Autodesk Fusion 360 part; units mm, degrees
(part 2 of 5)
  line L872 (126.5346, -132.5769) -> (126.5481, -132.5904)
  line L873 (126.5481, -132.5904) -> (126.55, -132.6)
  line L874 (126.55, -132.6) -> (126.55, -134.1)
  line L875 (126.55, -134.1) -> (126.5481, -134.1096)
  line L876 (126.5481, -134.1096) -> (126.5346, -134.1231)
  line L877 (126.5346, -134.1231) -> (126.525, -134.125)
  line L878 (126.525, -134.125) -> (121.125, -134.125)
  line L879 (121.125, -134.125) -> (121.1154, -134.1231)
  line L880 (121.1154, -134.1231) -> (121.1019, -134.1096)
  line L881 (121.1019, -134.1096) -> (121.1, -134.1)
  line L882 (121.1, -134.1) -> (121.1, -132.6)
  line L883 (121.1, -132.6) -> (121.1019, -132.5904)
  line L884 (121.1019, -132.5904) -> (121.1154, -132.5769)
  line L885 (121.1154, -132.5769) -> (121.125, -132.575)
  line L886 (121.125, -132.575) -> (126.525, -132.575)
  line L887 (126.525, -132.575) -> (126.5346, -132.5769)
  line L888 (121.15, -132.625) -> (121.15, -134.075)
  line L889 (121.15, -134.075) -> (126.5, -134.075)
  line L890 (126.5, -134.075) -> (126.5, -132.625)
  line L891 (126.5, -132.625) -> (121.15, -132.625)
  line L892 (62.5173, -130.6479) -> (62.5309, -130.6614)
  line L893 (62.5309, -130.6614) -> (62.5328, -130.671)
  line L894 (62.5328, -130.671) -> (62.5328, -132.1593)
  line L895 (62.5328, -132.1593) -> (62.5309, -132.1688)
  line L896 (62.5309, -132.1688) -> (62.5173, -132.1824)
  line L897 (62.5173, -132.1824) -> (62.5078, -132.1843)
  line L898 (62.5078, -132.1843) -> (61.0195, -132.1843)
  line L899 (61.0195, -132.1843) -> (61.0099, -132.1824)
  line L900 (61.0099, -132.1824) -> (60.9964, -132.1688)
  line L901 (60.9964, -132.1688) -> (60.9945, -132.1593)
  line L902 (60.9945, -132.1593) -> (60.9945, -130.671)
  line L903 (60.9945, -130.671) -> (60.9964, -130.6614)
  line L904 (60.9964, -130.6614) -> (61.0099, -130.6479)
  line L905 (61.0099, -130.6479) -> (61.0195, -130.646)
  line L906 (61.0195, -130.646) -> (62.5078, -130.646)
  line L907 (62.5078, -130.646) -> (62.5173, -130.6479)
  line L908 (61.0445, -130.696) -> (61.0445, -132.1343)
  line L909 (61.0445, -132.1343) -> (62.4828, -132.1343)
  line L910 (62.4828, -132.1343) -> (62.4828, -130.696)
  line L911 (62.4828, -130.696) -> (61.0445, -130.696)
  line L912 (67.5775, -130.6479) -> (67.591, -130.6614)
  line L913 (67.591, -130.6614) -> (67.5929, -130.671)
  line L914 (67.5929, -130.671) -> (67.5929, -132.1593)
  line L915 (67.5929, -132.1593) -> (67.591, -132.1688)
  line L916 (67.591, -132.1688) -> (67.5775, -132.1824)
  line L917 (67.5775, -132.1824) -> (67.5679, -132.1843)
  line L918 (67.5679, -132.1843) -> (66.0796, -132.1843)
  line L919 (66.0796, -132.1843) -> (66.0701, -132.1824)
  line L920 (66.0701, -132.1824) -> (66.0565, -132.1688)
  line L921 (66.0565, -132.1688) -> (66.0546, -132.1593)
  line L922 (66.0546, -132.1593) -> (66.0546, -130.671)
  line L923 (66.0546, -130.671) -> (66.0565, -130.6614)
  line L924 (66.0565, -130.6614) -> (66.0701, -130.6479)
  line L925 (66.0701, -130.6479) -> (66.0796, -130.646)
  line L926 (66.0796, -130.646) -> (67.5679, -130.646)
  line L927 (67.5679, -130.646) -> (67.5775, -130.6479)
  line L928 (66.1046, -130.696) -> (66.1046, -132.1343)
  line L929 (66.1046, -132.1343) -> (67.5429, -132.1343)
  line L930 (67.5429, -132.1343) -> (67.5429, -130.696)
  line L931 (67.5429, -130.696) -> (66.1046, -130.696)
  line L932 (93.1758, -121.4205) -> (93.1894, -121.4341)
  line L933 (93.1894, -121.4341) -> (93.1913, -121.4436)
  line L934 (93.1913, -121.4436) -> (93.1913, -125.0155)
  line L935 (93.1913, -125.0155) -> (93.1894, -125.0251)
  line L936 (93.1894, -125.0251) -> (93.1758, -125.0386)
  line L937 (93.1758, -125.0386) -> (93.1663, -125.0405)
  line L938 (93.1663, -125.0405) -> (90.81, -125.0405)
  line L939 (90.81, -125.0405) -> (90.81, -125.9085)
  line L940 (90.81, -125.9085) -> (90.8081, -125.918)
  line L941 (90.8081, -125.918) -> (90.7946, -125.9316)
  line L942 (90.7946, -125.9316) -> (90.785, -125.9335)
  line L943 (90.785, -125.9335) -> (88.1311, -125.9335)
  line L944 (88.1311, -125.9335) -> (88.1311, -129.778)
  line L945 (88.1311, -129.778) -> (88.1311, -130.9686)
  line L946 (88.1311, -130.9686) -> (88.1292, -130.9782)
  line L947 (88.1292, -130.9782) -> (88.1157, -130.9917)
  line L948 (88.1157, -130.9917) -> (88.1061, -130.9936)
  line L949 (88.1061, -130.9936) -> (83.6413, -130.9936)
  line L950 (83.6413, -130.9936) -> (83.3436, -130.9936)
  line L951 (83.3436, -130.9936) -> (83.334, -130.9917)
  line L952 (83.334, -130.9917) -> (83.3205, -130.9782)
  line L953 (83.3205, -130.9782) -> (83.3186, -130.9686)
  line L954 (83.3186, -130.9686) -> (83.3186, -128.0171)
  line L955 (83.3186, -128.0171) -> (81.8803, -128.0171)
  line L956 (81.8803, -128.0171) -> (81.8803, -129.778)
  line L957 (81.8803, -129.778) -> (81.8784, -129.7876)
  line L958 (81.8784, -129.7876) -> (81.8649, -129.8011)
  line L959 (81.8649, -129.8011) -> (81.8553, -129.803)
  line L960 (81.8553, -129.803) -> (79.4741, -129.803)
  line L961 (79.4741, -129.803) -> (79.4645, -129.8011)
  line L962 (79.4645, -129.8011) -> (79.451, -129.7876)
  line L963 (79.451, -129.7876) -> (79.4491, -129.778)
  line L964 (79.4491, -129.778) -> (79.4491, -127.7194)
  line L965 (79.4491, -127.7194) -> (77.0928, -127.7194)
  line L966 (77.0928, -127.7194) -> (77.0833, -127.7175)
  line L967 (77.0833, -127.7175) -> (77.0697, -127.704)
  line L968 (77.0697, -127.704) -> (77.0678, -127.6944)
  line L969 (77.0678, -127.6944) -> (77.0678, -124.4202)
  line L970 (77.0678, -124.4202) -> (77.0697, -124.4106)
  line L971 (77.0697, -124.4106) -> (77.0833, -124.3971)
  line L972 (77.0833, -124.3971) -> (77.0928, -124.3952)
  line L973 (77.0928, -124.3952) -> (79.4491, -124.3952)
  line L974 (79.4491, -124.3952) -> (79.4491, -121.4436)
  line L975 (79.4491, -121.4436) -> (79.451, -121.4341)
  line L976 (79.451, -121.4341) -> (79.4645, -121.4205)
  line L977 (79.4645, -121.4205) -> (79.4741, -121.4186)
  line L978 (79.4741, -121.4186) -> (93.1663, -121.4186)
  line L979 (93.1663, -121.4186) -> (93.1758, -121.4205)
  line L980 (79.4991, -121.4686) -> (79.4991, -124.4202)
  line L981 (79.4991, -124.4202) -> (79.4972, -124.4298)
  line L982 (79.4972, -124.4298) -> (79.4836, -124.4433)
  line L983 (79.4836, -124.4433) -> (79.4741, -124.4452)
  line L984 (79.4741, -124.4452) -> (77.1178, -124.4452)
  line L985 (77.1178, -124.4452) -> (77.1178, -127.6694)
  line L986 (77.1178, -127.6694) -> (79.4741, -127.6694)
  line L987 (79.4741, -127.6694) -> (79.4836, -127.6713)
  line L988 (79.4836, -127.6713) -> (79.4972, -127.6848)
  line L989 (79.4972, -127.6848) -> (79.4991, -127.6944)
  line L990 (79.4991, -127.6944) -> (79.4991, -129.753)
  line L991 (79.4991, -129.753) -> (81.8303, -129.753)
  line L992 (81.8303, -129.753) -> (81.8303, -127.9921)
  line L993 (81.8303, -127.9921) -> (81.8322, -127.9825)
  line L994 (81.8322, -127.9825) -> (81.8458, -127.969)
  line L995 (81.8458, -127.969) -> (81.8553, -127.9671)
  line L996 (81.8553, -127.9671) -> (83.3436, -127.9671)
  line L997 (83.3436, -127.9671) -> (83.3532, -127.969)
  line L998 (83.3532, -127.969) -> (83.3667, -127.9825)
  line L999 (83.3667, -127.9825) -> (83.3686, -127.9921)
  line L1000 (83.3686, -127.9921) -> (83.3686, -130.9436)
  line L1001 (83.3686, -130.9436) -> (83.6413, -130.9436)
  line L1002 (83.6413, -130.9436) -> (88.0811, -130.9436)
  line L1003 (88.0811, -130.9436) -> (88.0811, -129.778)
  line L1004 (88.0811, -129.778) -> (88.0811, -125.9085)
  line L1005 (88.0811, -125.9085) -> (88.083, -125.8989)
  line L1006 (88.083, -125.8989) -> (88.0965, -125.8854)
  line L1007 (88.0965, -125.8854) -> (88.1061, -125.8835)
  line L1008 (88.1061, -125.8835) -> (90.76, -125.8835)
  line L1009 (90.76, -125.8835) -> (90.76, -125.0155)
  line L1010 (90.76, -125.0155) -> (90.7619, -125.0059)
  line L1011 (90.7619, -125.0059) -> (90.7754, -124.9924)
  line L1012 (90.7754, -124.9924) -> (90.785, -124.9905)
  line L1013 (90.785, -124.9905) -> (93.1413, -124.9905)
  line L1014 (93.1413, -124.9905) -> (93.1413, -121.4686)
  line L1015 (93.1413, -121.4686) -> (79.4991, -121.4686)
  line L1016 (112.2258, -121.4205) -> (112.2394, -121.4341)
  line L1017 (112.2394, -121.4341) -> (112.2413, -121.4436)
  line L1018 (112.2413, -121.4436) -> (112.2413, -125.0155)
  line L1019 (112.2413, -125.0155) -> (112.2394, -125.0251)
  line L1020 (112.2394, -125.0251) -> (112.2258, -125.0386)
  line L1021 (112.2258, -125.0386) -> (112.2163, -125.0405)
  line L1022 (112.2163, -125.0405) -> (109.86, -125.0405)
  line L1023 (109.86, -125.0405) -> (109.86, -125.9085)
  line L1024 (109.86, -125.9085) -> (109.8581, -125.918)
  line L1025 (109.8581, -125.918) -> (109.8446, -125.9316)
  line L1026 (109.8446, -125.9316) -> (109.835, -125.9335)
  line L1027 (109.835, -125.9335) -> (107.1811, -125.9335)
  line L1028 (107.1811, -125.9335) -> (107.1811, -129.778)
  line L1029 (107.1811, -129.778) -> (107.1811, -130.9686)
  line L1030 (107.1811, -130.9686) -> (107.1792, -130.9782)
  line L1031 (107.1792, -130.9782) -> (107.1657, -130.9917)
  line L1032 (107.1657, -130.9917) -> (107.1561, -130.9936)
  line L1033 (107.1561, -130.9936) -> (102.6913, -130.9936)
  line L1034 (102.6913, -130.9936) -> (102.3936, -130.9936)
  line L1035 (102.3936, -130.9936) -> (102.384, -130.9917)
  line L1036 (102.384, -130.9917) -> (102.3705, -130.9782)
  line L1037 (102.3705, -130.9782) -> (102.3686, -130.9686)
  line L1038 (102.3686, -130.9686) -> (102.3686, -128.0171)
  line L1039 (102.3686, -128.0171) -> (100.9303, -128.0171)
  line L1040 (100.9303, -128.0171) -> (100.9303, -129.778)
  line L1041 (100.9303, -129.778) -> (100.9284, -129.7876)
  line L1042 (100.9284, -129.7876) -> (100.9149, -129.8011)
  line L1043 (100.9149, -129.8011) -> (100.9053, -129.803)
  line L1044 (100.9053, -129.803) -> (98.5241, -129.803)
  line L1045 (98.5241, -129.803) -> (98.5145, -129.8011)
  line L1046 (98.5145, -129.8011) -> (98.501, -129.7876)
  line L1047 (98.501, -129.7876) -> (98.4991, -129.778)
  line L1048 (98.4991, -129.778) -> (98.4991, -127.7194)
  line L1049 (98.4991, -127.7194) -> (96.1428, -127.7194)
  line L1050 (96.1428, -127.7194) -> (96.1333, -127.7175)
  line L1051 (96.1333, -127.7175) -> (96.1197, -127.704)
  line L1052 (96.1197, -127.704) -> (96.1178, -127.6944)
  line L1053 (96.1178, -127.6944) -> (96.1178, -124.4202)
  line L1054 (96.1178, -124.4202) -> (96.1197, -124.4106)
  line L1055 (96.1197, -124.4106) -> (96.1333, -124.3971)
  line L1056 (96.1333, -124.3971) -> (96.1428, -124.3952)
  line L1057 (96.1428, -124.3952) -> (98.4991, -124.3952)
  line L1058 (98.4991, -124.3952) -> (98.4991, -121.4436)
  line L1059 (98.4991, -121.4436) -> (98.501, -121.4341)
  line L1060 (98.501, -121.4341) -> (98.5145, -121.4205)
  line L1061 (98.5145, -121.4205) -> (98.5241, -121.4186)
  line L1062 (98.5241, -121.4186) -> (112.2163, -121.4186)
  line L1063 (112.2163, -121.4186) -> (112.2258, -121.4205)
  line L1064 (98.5491, -121.4686) -> (98.5491, -124.4202)
  line L1065 (98.5491, -124.4202) -> (98.5472, -124.4298)
  line L1066 (98.5472, -124.4298) -> (98.5336, -124.4433)
  line L1067 (98.5336, -124.4433) -> (98.5241, -124.4452)
  line L1068 (98.5241, -124.4452) -> (96.1678, -124.4452)
  line L1069 (96.1678, -124.4452) -> (96.1678, -127.6694)
  line L1070 (96.1678, -127.6694) -> (98.5241, -127.6694)
  line L1071 (98.5241, -127.6694) -> (98.5336, -127.6713)
  line L1072 (98.5336, -127.6713) -> (98.5472, -127.6848)
  line L1073 (98.5472, -127.6848) -> (98.5491, -127.6944)
  line L1074 (98.5491, -127.6944) -> (98.5491, -129.753)
  line L1075 (98.5491, -129.753) -> (100.8803, -129.753)
  line L1076 (100.8803, -129.753) -> (100.8803, -127.9921)
  line L1077 (100.8803, -127.9921) -> (100.8822, -127.9825)
  line L1078 (100.8822, -127.9825) -> (100.8958, -127.969)
  line L1079 (100.8958, -127.969) -> (100.9053, -127.9671)
  line L1080 (100.9053, -127.9671) -> (102.3936, -127.9671)
  line L1081 (102.3936, -127.9671) -> (102.4032, -127.969)
  line L1082 (102.4032, -127.969) -> (102.4167, -127.9825)
  line L1083 (102.4167, -127.9825) -> (102.4186, -127.9921)
  line L1084 (102.4186, -127.9921) -> (102.4186, -130.9436)
  line L1085 (102.4186, -130.9436) -> (102.6913, -130.9436)
  line L1086 (102.6913, -130.9436) -> (107.1311, -130.9436)
  line L1087 (107.1311, -130.9436) -> (107.1311, -129.778)
  line L1088 (107.1311, -129.778) -> (107.1311, -125.9085)
  line L1089 (107.1311, -125.9085) -> (107.133, -125.8989)
  line L1090 (107.133, -125.8989) -> (107.1465, -125.8854)
  line L1091 (107.1465, -125.8854) -> (107.1561, -125.8835)
  line L1092 (107.1561, -125.8835) -> (109.81, -125.8835)
  line L1093 (109.81, -125.8835) -> (109.81, -125.0155)
  line L1094 (109.81, -125.0155) -> (109.8119, -125.0059)
  line L1095 (109.8119, -125.0059) -> (109.8254, -124.9924)
  line L1096 (109.8254, -124.9924) -> (109.835, -124.9905)
  line L1097 (109.835, -124.9905) -> (112.1913, -124.9905)
  line L1098 (112.1913, -124.9905) -> (112.1913, -121.4686)
  line L1099 (112.1913, -121.4686) -> (98.5491, -121.4686)
  line L1100 (131.2758, -121.4205) -> (131.2894, -121.4341)
  line L1101 (131.2894, -121.4341) -> (131.2913, -121.4436)
  line L1102 (131.2913, -121.4436) -> (131.2913, -125.0155)
  line L1103 (131.2913, -125.0155) -> (131.2894, -125.0251)
  line L1104 (131.2894, -125.0251) -> (131.2758, -125.0386)
  line L1105 (131.2758, -125.0386) -> (131.2663, -125.0405)
  line L1106 (131.2663, -125.0405) -> (128.91, -125.0405)
  line L1107 (128.91, -125.0405) -> (128.91, -125.9085)
  line L1108 (128.91, -125.9085) -> (128.9081, -125.918)
  line L1109 (128.9081, -125.918) -> (128.8946, -125.9316)
  line L1110 (128.8946, -125.9316) -> (128.885, -125.9335)
  line L1111 (128.885, -125.9335) -> (126.2311, -125.9335)
  line L1112 (126.2311, -125.9335) -> (126.2311, -129.778)
  line L1113 (126.2311, -129.778) -> (126.2311, -130.9686)
  line L1114 (126.2311, -130.9686) -> (126.2292, -130.9782)
  line L1115 (126.2292, -130.9782) -> (126.2157, -130.9917)
  line L1116 (126.2157, -130.9917) -> (126.2061, -130.9936)
  line L1117 (126.2061, -130.9936) -> (121.7413, -130.9936)
  line L1118 (121.7413, -130.9936) -> (121.4436, -130.9936)
  line L1119 (121.4436, -130.9936) -> (121.434, -130.9917)
  line L1120 (121.434, -130.9917) -> (121.4205, -130.9782)
  line L1121 (121.4205, -130.9782) -> (121.4186, -130.9686)
  line L1122 (121.4186, -130.9686) -> (121.4186, -128.0171)
  line L1123 (121.4186, -128.0171) -> (119.9803, -128.0171)
  line L1124 (119.9803, -128.0171) -> (119.9803, -129.778)
  line L1125 (119.9803, -129.778) -> (119.9784, -129.7876)
  line L1126 (119.9784, -129.7876) -> (119.9649, -129.8011)
  line L1127 (119.9649, -129.8011) -> (119.9553, -129.803)
  line L1128 (119.9553, -129.803) -> (117.5741, -129.803)
  line L1129 (117.5741, -129.803) -> (117.5645, -129.8011)
  line L1130 (117.5645, -129.8011) -> (117.551, -129.7876)
  line L1131 (117.551, -129.7876) -> (117.5491, -129.778)
  line L1132 (117.5491, -129.778) -> (117.5491, -127.7194)
  line L1133 (117.5491, -127.7194) -> (115.1928, -127.7194)
  line L1134 (115.1928, -127.7194) -> (115.1833, -127.7175)
  line L1135 (115.1833, -127.7175) -> (115.1697, -127.704)
  line L1136 (115.1697, -127.704) -> (115.1678, -127.6944)
  line L1137 (115.1678, -127.6944) -> (115.1678, -124.4202)
  line L1138 (115.1678, -124.4202) -> (115.1697, -124.4106)
  line L1139 (115.1697, -124.4106) -> (115.1833, -124.3971)
  line L1140 (115.1833, -124.3971) -> (115.1928, -124.3952)
  line L1141 (115.1928, -124.3952) -> (117.5491, -124.3952)
  line L1142 (117.5491, -124.3952) -> (117.5491, -121.4436)
  line L1143 (117.5491, -121.4436) -> (117.551, -121.4341)
  line L1144 (117.551, -121.4341) -> (117.5645, -121.4205)
  line L1145 (117.5645, -121.4205) -> (117.5741, -121.4186)
  line L1146 (117.5741, -121.4186) -> (131.2663, -121.4186)
  line L1147 (131.2663, -121.4186) -> (131.2758, -121.4205)
  line L1148 (117.5991, -121.4686) -> (117.5991, -124.4202)
  line L1149 (117.5991, -124.4202) -> (117.5972, -124.4298)
  line L1150 (117.5972, -124.4298) -> (117.5836, -124.4433)
  line L1151 (117.5836, -124.4433) -> (117.5741, -124.4452)
  line L1152 (117.5741, -124.4452) -> (115.2178, -124.4452)
  line L1153 (115.2178, -124.4452) -> (115.2178, -127.6694)
  line L1154 (115.2178, -127.6694) -> (117.5741, -127.6694)
  line L1155 (117.5741, -127.6694) -> (117.5836, -127.6713)
  line L1156 (117.5836, -127.6713) -> (117.5972, -127.6848)
  line L1157 (117.5972, -127.6848) -> (117.5991, -127.6944)
  line L1158 (117.5991, -127.6944) -> (117.5991, -129.753)
  line L1159 (117.5991, -129.753) -> (119.9303, -129.753)
  line L1160 (119.9303, -129.753) -> (119.9303, -127.9921)
  line L1161 (119.9303, -127.9921) -> (119.9322, -127.9825)
  line L1162 (119.9322, -127.9825) -> (119.9458, -127.969)
  line L1163 (119.9458, -127.969) -> (119.9553, -127.9671)
  line L1164 (119.9553, -127.9671) -> (121.4436, -127.9671)
  line L1165 (121.4436, -127.9671) -> (121.4532, -127.969)
  line L1166 (121.4532, -127.969) -> (121.4667, -127.9825)
  line L1167 (121.4667, -127.9825) -> (121.4686, -127.9921)
  line L1168 (121.4686, -127.9921) -> (121.4686, -130.9436)
  line L1169 (121.4686, -130.9436) -> (121.7413, -130.9436)
  line L1170 (121.7413, -130.9436) -> (126.1811, -130.9436)
  line L1171 (126.1811, -130.9436) -> (126.1811, -129.778)
  line L1172 (126.1811, -129.778) -> (126.1811, -125.9085)
  line L1173 (126.1811, -125.9085) -> (126.183, -125.8989)
  line L1174 (126.183, -125.8989) -> (126.1965, -125.8854)
  line L1175 (126.1965, -125.8854) -> (126.2061, -125.8835)
  line L1176 (126.2061, -125.8835) -> (128.86, -125.8835)
  line L1177 (128.86, -125.8835) -> (128.86, -125.0155)
  line L1178 (128.86, -125.0155) -> (128.8619, -125.0059)
  line L1179 (128.8619, -125.0059) -> (128.8754, -124.9924)
  line L1180 (128.8754, -124.9924) -> (128.885, -124.9905)
  line L1181 (128.885, -124.9905) -> (131.2413, -124.9905)
  line L1182 (131.2413, -124.9905) -> (131.2413, -121.4686)
  line L1183 (131.2413, -121.4686) -> (117.5991, -121.4686)
  line L1184 (90.9961, -127.3902) -> (91.2008, -127.4451)
  line L1185 (91.2008, -127.4451) -> (91.3928, -127.5346)
  line L1186 (91.3928, -127.5346) -> (91.5664, -127.6562)
  line L1187 (91.5664, -127.6562) -> (91.7162, -127.806)
  line L1188 (91.7162, -127.806) -> (91.8378, -127.9796)
  line L1189 (91.8378, -127.9796) -> (91.9273, -128.1716)
  line L1190 (91.9273, -128.1716) -> (91.9822, -128.3763)
  line L1191 (91.9822, -128.3763) -> (92.0006, -128.5874)
  line L1192 (92.0006, -128.5874) -> (91.9822, -128.7985)
  line L1193 (91.9822, -128.7985) -> (91.9273, -129.0031)
  line L1194 (91.9273, -129.0031) -> (91.8378, -129.1952)
  line L1195 (91.8378, -129.1952) -> (91.7162, -129.3688)
  line L1196 (91.7162, -129.3688) -> (91.5664, -129.5186)
  line L1197 (91.5664, -129.5186) -> (91.3928, -129.6401)
  line L1198 (91.3928, -129.6401) -> (91.2008, -129.7297)
  line L1199 (91.2008, -129.7297) -> (90.9961, -129.7845)
  line L1200 (90.9961, -129.7845) -> (90.785, -129.803)
  line L1201 (90.785, -129.803) -> (90.5739, -129.7845)
  line L1202 (90.5739, -129.7845) -> (90.3692, -129.7297)
  line L1203 (90.3692, -129.7297) -> (90.1772, -129.6401)
  line L1204 (90.1772, -129.6401) -> (90.0036, -129.5186)
  line L1205 (90.0036, -129.5186) -> (89.8538, -129.3688)
  line L1206 (89.8538, -129.3688) -> (89.7322, -129.1952)
  line L1207 (89.7322, -129.1952) -> (89.6427, -129.0031)
  line L1208 (89.6427, -129.0031) -> (89.5879, -128.7985)
  line L1209 (89.5879, -128.7985) -> (89.5694, -128.5874)
  line L1210 (89.5694, -128.5874) -> (89.5879, -128.3763)
  line L1211 (89.5879, -128.3763) -> (89.6427, -128.1716)
  line L1212 (89.6427, -128.1716) -> (89.7322, -127.9796)
  line L1213 (89.7322, -127.9796) -> (89.8538, -127.806)
  line L1214 (89.8538, -127.806) -> (90.0036, -127.6562)
  line L1215 (90.0036, -127.6562) -> (90.1772, -127.5346)
  line L1216 (90.1772, -127.5346) -> (90.3692, -127.4451)
  line L1217 (90.3692, -127.4451) -> (90.5739, -127.3902)
  line L1218 (90.5739, -127.3902) -> (90.785, -127.3718)
  line L1219 (90.785, -127.3718) -> (90.9961, -127.3902)
  line L1220 (89.6343, -128.8025) -> (89.6934, -129.0103)
  line L1221 (89.6934, -129.0103) -> (89.7897, -129.2036)
  line L1222 (89.7897, -129.2036) -> (89.9199, -129.376)
  line L1223 (89.9199, -129.376) -> (90.0796, -129.5215)
  line L1224 (90.0796, -129.5215) -> (90.2632, -129.6353)
  line L1225 (90.2632, -129.6353) -> (90.4647, -129.7133)
  line L1226 (90.4647, -129.7133) -> (90.677, -129.753)
  line L1227 (90.677, -129.753) -> (90.893, -129.753)
  line L1228 (90.893, -129.753) -> (91.1054, -129.7133)
  line L1229 (91.1054, -129.7133) -> (91.3068, -129.6353)
  line L1230 (91.3068, -129.6353) -> (91.4905, -129.5215)
  line L1231 (91.4905, -129.5215) -> (91.6501, -129.376)
  line L1232 (91.6501, -129.376) -> (91.7803, -129.2036)
  line L1233 (91.7803, -129.2036) -> (91.8766, -129.0103)
  line L1234 (91.8766, -129.0103) -> (91.9357, -128.8025)
  line L1235 (91.9357, -128.8025) -> (91.9556, -128.5874)
  line L1236 (91.9556, -128.5874) -> (91.9357, -128.3723)
  line L1237 (91.9357, -128.3723) -> (91.8766, -128.1645)
  line L1238 (91.8766, -128.1645) -> (91.7803, -127.9711)
  line L1239 (91.7803, -127.9711) -> (91.6501, -127.7987)
  line L1240 (91.6501, -127.7987) -> (91.4905, -127.6532)
  line L1241 (91.4905, -127.6532) -> (91.3068, -127.5395)
  line L1242 (91.3068, -127.5395) -> (91.1054, -127.4614)
  line L1243 (91.1054, -127.4614) -> (90.893, -127.4218)
  line L1244 (90.893, -127.4218) -> (90.677, -127.4218)
  line L1245 (90.677, -127.4218) -> (90.4647, -127.4614)
  line L1246 (90.4647, -127.4614) -> (90.2632, -127.5395)
  line L1247 (90.2632, -127.5395) -> (90.0796, -127.6532)
  line L1248 (90.0796, -127.6532) -> (89.9199, -127.7987)
  line L1249 (89.9199, -127.7987) -> (89.7897, -127.9711)
  line L1250 (89.7897, -127.9711) -> (89.6934, -128.1645)
  line L1251 (89.6934, -128.1645) -> (89.6343, -128.3723)
  line L1252 (89.6343, -128.3723) -> (89.6144, -128.5874)
  line L1253 (89.6144, -128.5874) -> (89.6343, -128.8025)
  line L1254 (110.0461, -127.3902) -> (110.2508, -127.4451)
  line L1255 (110.2508, -127.4451) -> (110.4428, -127.5346)
  line L1256 (110.4428, -127.5346) -> (110.6164, -127.6562)
  line L1257 (110.6164, -127.6562) -> (110.7662, -127.806)
  line L1258 (110.7662, -127.806) -> (110.8878, -127.9796)
  line L1259 (110.8878, -127.9796) -> (110.9773, -128.1716)
  line L1260 (110.9773, -128.1716) -> (111.0322, -128.3763)
  line L1261 (111.0322, -128.3763) -> (111.0506, -128.5874)
  line L1262 (111.0506, -128.5874) -> (111.0322, -128.7985)
  line L1263 (111.0322, -128.7985) -> (110.9773, -129.0031)
  line L1264 (110.9773, -129.0031) -> (110.8878, -129.1952)
  line L1265 (110.8878, -129.1952) -> (110.7662, -129.3688)
  line L1266 (110.7662, -129.3688) -> (110.6164, -129.5186)
  line L1267 (110.6164, -129.5186) -> (110.4428, -129.6401)
  line L1268 (110.4428, -129.6401) -> (110.2508, -129.7297)
  line L1269 (110.2508, -129.7297) -> (110.0461, -129.7845)
  line L1270 (110.0461, -129.7845) -> (109.835, -129.803)
  line L1271 (109.835, -129.803) -> (109.6239, -129.7845)
  line L1272 (109.6239, -129.7845) -> (109.4192, -129.7297)
  line L1273 (109.4192, -129.7297) -> (109.2272, -129.6401)
  line L1274 (109.2272, -129.6401) -> (109.0536, -129.5186)
  line L1275 (109.0536, -129.5186) -> (108.9038, -129.3688)
  line L1276 (108.9038, -129.3688) -> (108.7822, -129.1952)
  line L1277 (108.7822, -129.1952) -> (108.6927, -129.0031)
  line L1278 (108.6927, -129.0031) -> (108.6379, -128.7985)
  line L1279 (108.6379, -128.7985) -> (108.6194, -128.5874)
  line L1280 (108.6194, -128.5874) -> (108.6379, -128.3763)
  line L1281 (108.6379, -128.3763) -> (108.6927, -128.1716)
  line L1282 (108.6927, -128.1716) -> (108.7822, -127.9796)
  line L1283 (108.7822, -127.9796) -> (108.9038, -127.806)
  line L1284 (108.9038, -127.806) -> (109.0536, -127.6562)
  line L1285 (109.0536, -127.6562) -> (109.2272, -127.5346)
  line L1286 (109.2272, -127.5346) -> (109.4192, -127.4451)
  line L1287 (109.4192, -127.4451) -> (109.6239, -127.3902)
  line L1288 (109.6239, -127.3902) -> (109.835, -127.3718)
  line L1289 (109.835, -127.3718) -> (110.0461, -127.3902)
  line L1290 (108.6843, -128.8025) -> (108.7434, -129.0103)
  line L1291 (108.7434, -129.0103) -> (108.8397, -129.2036)
  line L1292 (108.8397, -129.2036) -> (108.9699, -129.376)
  line L1293 (108.9699, -129.376) -> (109.1296, -129.5215)
  line L1294 (109.1296, -129.5215) -> (109.3132, -129.6353)
  line L1295 (109.3132, -129.6353) -> (109.5147, -129.7133)
  line L1296 (109.5147, -129.7133) -> (109.727, -129.753)
  line L1297 (109.727, -129.753) -> (109.943, -129.753)
  line L1298 (109.943, -129.753) -> (110.1554, -129.7133)
  line L1299 (110.1554, -129.7133) -> (110.3568, -129.6353)
  line L1300 (110.3568, -129.6353) -> (110.5405, -129.5215)
  line L1301 (110.5405, -129.5215) -> (110.7001, -129.376)
  line L1302 (110.7001, -129.376) -> (110.8303, -129.2036)
  line L1303 (110.8303, -129.2036) -> (110.9266, -129.0103)
  line L1304 (110.9266, -129.0103) -> (110.9857, -128.8025)
  line L1305 (110.9857, -128.8025) -> (111.0056, -128.5874)
  line L1306 (111.0056, -128.5874) -> (110.9857, -128.3723)
  line L1307 (110.9857, -128.3723) -> (110.9266, -128.1645)
  line L1308 (110.9266, -128.1645) -> (110.8303, -127.9711)
  line L1309 (110.8303, -127.9711) -> (110.7001, -127.7987)
  line L1310 (110.7001, -127.7987) -> (110.5405, -127.6532)
  line L1311 (110.5405, -127.6532) -> (110.3568, -127.5395)
  line L1312 (110.3568, -127.5395) -> (110.1554, -127.4614)
  line L1313 (110.1554, -127.4614) -> (109.943, -127.4218)
  line L1314 (109.943, -127.4218) -> (109.727, -127.4218)
  line L1315 (109.727, -127.4218) -> (109.5147, -127.4614)
  line L1316 (109.5147, -127.4614) -> (109.3132, -127.5395)
  line L1317 (109.3132, -127.5395) -> (109.1296, -127.6532)
  line L1318 (109.1296, -127.6532) -> (108.9699, -127.7987)
  line L1319 (108.9699, -127.7987) -> (108.8397, -127.9711)
  line L1320 (108.8397, -127.9711) -> (108.7434, -128.1645)
  line L1321 (108.7434, -128.1645) -> (108.6843, -128.3723)
  line L1322 (108.6843, -128.3723) -> (108.6644, -128.5874)
  line L1323 (108.6644, -128.5874) -> (108.6843, -128.8025)
  line L1324 (129.0961, -127.3902) -> (129.3008, -127.4451)
  line L1325 (129.3008, -127.4451) -> (129.4928, -127.5346)
  line L1326 (129.4928, -127.5346) -> (129.6664, -127.6562)
  line L1327 (129.6664, -127.6562) -> (129.8162, -127.806)
  line L1328 (129.8162, -127.806) -> (129.9378, -127.9796)
  line L1329 (129.9378, -127.9796) -> (130.0273, -128.1716)
  line L1330 (130.0273, -128.1716) -> (130.0822, -128.3763)
  line L1331 (130.0822, -128.3763) -> (130.1006, -128.5874)
  line L1332 (130.1006, -128.5874) -> (130.0822, -128.7985)
  line L1333 (130.0822, -128.7985) -> (130.0273, -129.0031)
  line L1334 (130.0273, -129.0031) -> (129.9378, -129.1952)
  line L1335 (129.9378, -129.1952) -> (129.8162, -129.3688)
  line L1336 (129.8162, -129.3688) -> (129.6664, -129.5186)
  line L1337 (129.6664, -129.5186) -> (129.4928, -129.6401)
  line L1338 (129.4928, -129.6401) -> (129.3008, -129.7297)
  line L1339 (129.3008, -129.7297) -> (129.0961, -129.7845)
  line L1340 (129.0961, -129.7845) -> (128.885, -129.803)
  line L1341 (128.885, -129.803) -> (128.6739, -129.7845)
  line L1342 (128.6739, -129.7845) -> (128.4692, -129.7297)
  line L1343 (128.4692, -129.7297) -> (128.2772, -129.6401)
  line L1344 (128.2772, -129.6401) -> (128.1036, -129.5186)
  line L1345 (128.1036, -129.5186) -> (127.9538, -129.3688)
  line L1346 (127.9538, -129.3688) -> (127.8322, -129.1952)
  line L1347 (127.8322, -129.1952) -> (127.7427, -129.0031)
  line L1348 (127.7427, -129.0031) -> (127.6879, -128.7985)
  line L1349 (127.6879, -128.7985) -> (127.6694, -128.5874)
  line L1350 (127.6694, -128.5874) -> (127.6879, -128.3763)
  line L1351 (127.6879, -128.3763) -> (127.7427, -128.1716)
  line L1352 (127.7427, -128.1716) -> (127.8322, -127.9796)
  line L1353 (127.8322, -127.9796) -> (127.9538, -127.806)
  line L1354 (127.9538, -127.806) -> (128.1036, -127.6562)
  line L1355 (128.1036, -127.6562) -> (128.2772, -127.5346)
  line L1356 (128.2772, -127.5346) -> (128.4692, -127.4451)
  line L1357 (128.4692, -127.4451) -> (128.6739, -127.3902)
  line L1358 (128.6739, -127.3902) -> (128.885, -127.3718)
  line L1359 (128.885, -127.3718) -> (129.0961, -127.3902)
  line L1360 (127.7343, -128.8025) -> (127.7934, -129.0103)
  line L1361 (127.7934, -129.0103) -> (127.8897, -129.2036)
  line L1362 (127.8897, -129.2036) -> (128.0199, -129.376)
  line L1363 (128.0199, -129.376) -> (128.1796, -129.5215)
  line L1364 (128.1796, -129.5215) -> (128.3632, -129.6353)
  line L1365 (128.3632, -129.6353) -> (128.5647, -129.7133)
  line L1366 (128.5647, -129.7133) -> (128.777, -129.753)
  line L1367 (128.777, -129.753) -> (128.993, -129.753)
  line L1368 (128.993, -129.753) -> (129.2054, -129.7133)
  line L1369 (129.2054, -129.7133) -> (129.4068, -129.6353)
  line L1370 (129.4068, -129.6353) -> (129.5905, -129.5215)
  line L1371 (129.5905, -129.5215) -> (129.7501, -129.376)
  line L1372 (129.7501, -129.376) -> (129.8803, -129.2036)
  line L1373 (129.8803, -129.2036) -> (129.9766, -129.0103)
  line L1374 (129.9766, -129.0103) -> (130.0357, -128.8025)
  line L1375 (130.0357, -128.8025) -> (130.0556, -128.5874)
  line L1376 (130.0556, -128.5874) -> (130.0357, -128.3723)
  line L1377 (130.0357, -128.3723) -> (129.9766, -128.1645)
  line L1378 (129.9766, -128.1645) -> (129.8803, -127.9711)
  line L1379 (129.8803, -127.9711) -> (129.7501, -127.7987)
  line L1380 (129.7501, -127.7987) -> (129.5905, -127.6532)
  line L1381 (129.5905, -127.6532) -> (129.4068, -127.5395)
  line L1382 (129.4068, -127.5395) -> (129.2054, -127.4614)
  line L1383 (129.2054, -127.4614) -> (128.993, -127.4218)
  line L1384 (128.993, -127.4218) -> (128.777, -127.4218)
  line L1385 (128.777, -127.4218) -> (128.5647, -127.4614)
  line L1386 (128.5647, -127.4614) -> (128.3632, -127.5395)
  line L1387 (128.3632, -127.5395) -> (128.1796, -127.6532)
  line L1388 (128.1796, -127.6532) -> (128.0199, -127.7987)
  line L1389 (128.0199, -127.7987) -> (127.8897, -127.9711)
  line L1390 (127.8897, -127.9711) -> (127.7934, -128.1645)
  line L1391 (127.7934, -128.1645) -> (127.7343, -128.3723)
  line L1392 (127.7343, -128.3723) -> (127.7144, -128.5874)
  line L1393 (127.7144, -128.5874) -> (127.7343, -128.8025)
  line L1394 (67.0033, -127.8144) -> (67.0168, -127.8279)
  line L1395 (67.0168, -127.8279) -> (67.0187, -127.8375)
  line L1396 (67.0187, -127.8375) -> (67.0187, -129.3375)
  line L1397 (67.0187, -129.3375) -> (67.0168, -129.3471)
  line L1398 (67.0168, -129.3471) -> (67.0033, -129.3606)
  line L1399 (67.0033, -129.3606) -> (66.9938, -129.3625)
  line L1400 (66.9938, -129.3625) -> (61.5938, -129.3625)
  line L1401 (61.5938, -129.3625) -> (61.5842, -129.3606)
  line L1402 (61.5842, -129.3606) -> (61.5707, -129.3471)
  line L1403 (61.5707, -129.3471) -> (61.5688, -129.3375)
  line L1404 (61.5688, -129.3375) -> (61.5688, -127.8375)
  line L1405 (61.5688, -127.8375) -> (61.5707, -127.8279)
  line L1406 (61.5707, -127.8279) -> (61.5842, -127.8144)
  line L1407 (61.5842, -127.8144) -> (61.5938, -127.8125)
  line L1408 (61.5938, -127.8125) -> (66.9938, -127.8125)
  line L1409 (66.9938, -127.8125) -> (67.0033, -127.8144)
  line L1410 (61.6188, -127.8625) -> (61.6188, -129.3125)
  line L1411 (61.6188, -129.3125) -> (66.9688, -129.3125)
  line L1412 (66.9688, -129.3125) -> (66.9688, -127.8625)
  line L1413 (66.9688, -127.8625) -> (61.6187, -127.8625)
  line L1414 (67.8751, -115.4674) -> (67.8887, -115.4809)
  line L1415 (67.8887, -115.4809) -> (67.8906, -115.4905)
  line L1416 (67.8906, -115.4905) -> (67.8906, -116.6561)
  line L1417 (67.8906, -116.6561) -> (71.735, -116.6561)
  line L1418 (71.735, -116.6561) -> (71.7446, -116.658)
  line L1419 (71.7446, -116.658) -> (71.7581, -116.6716)
  line L1420 (71.7581, -116.6716) -> (71.76, -116.6811)
  line L1421 (71.76, -116.6811) -> (71.76, -120.253)
  line L1422 (71.76, -120.253) -> (71.7581, -120.2626)
  line L1423 (71.7581, -120.2626) -> (71.7446, -120.2761)
  line L1424 (71.7446, -120.2761) -> (71.735, -120.278)
  line L1425 (71.735, -120.278) -> (69.3788, -120.278)
  line L1426 (69.3788, -120.278) -> (69.3788, -121.146)
  line L1427 (69.3788, -121.146) -> (69.3769, -121.1555)
  line L1428 (69.3769, -121.1555) -> (69.3633, -121.1691)
  line L1429 (69.3633, -121.1691) -> (69.3538, -121.171)
  line L1430 (69.3538, -121.171) -> (66.6999, -121.171)
  line L1431 (66.6999, -121.171) -> (66.6999, -125.0155)
  line L1432 (66.6999, -125.0155) -> (66.6999, -126.2061)
  line L1433 (66.6999, -126.2061) -> (66.698, -126.2157)
  line L1434 (66.698, -126.2157) -> (66.6844, -126.2292)
  line L1435 (66.6844, -126.2292) -> (66.6749, -126.2311)
  line L1436 (66.6749, -126.2311) -> (62.21, -126.2311)
  line L1437 (62.21, -126.2311) -> (61.9124, -126.2311)
  line L1438 (61.9124, -126.2311) -> (61.9028, -126.2292)
  line L1439 (61.9028, -126.2292) -> (61.8893, -126.2157)
  line L1440 (61.8893, -126.2157) -> (61.8874, -126.2061)
  line L1441 (61.8874, -126.2061) -> (61.8874, -123.2546)
  line L1442 (61.8874, -123.2546) -> (60.4491, -123.2546)
  line L1443 (60.4491, -123.2546) -> (60.4491, -125.0155)
  line L1444 (60.4491, -125.0155) -> (60.4472, -125.0251)
  line L1445 (60.4472, -125.0251) -> (60.4336, -125.0386)
  line L1446 (60.4336, -125.0386) -> (60.4241, -125.0405)
  line L1447 (60.4241, -125.0405) -> (58.0678, -125.0405)
  line L1448 (58.0678, -125.0405) -> (58.0678, -125.6108)
  line L1449 (58.0678, -125.6108) -> (58.0659, -125.6204)
  line L1450 (58.0659, -125.6204) -> (58.0524, -125.6339)
  line L1451 (58.0524, -125.6339) -> (58.0428, -125.6358)
  line L1452 (58.0428, -125.6358) -> (55.364, -125.6358)
  line L1453 (55.364, -125.6358) -> (55.3544, -125.6339)
  line L1454 (55.3544, -125.6339) -> (55.3409, -125.6204)
  line L1455 (55.3409, -125.6204) -> (55.339, -125.6108)
  line L1456 (55.339, -125.6108) -> (55.339, -119.6577)
  line L1457 (55.339, -119.6577) -> (55.3409, -119.6481)
  line L1458 (55.3409, -119.6481) -> (55.3544, -119.6346)
  line L1459 (55.3544, -119.6346) -> (55.364, -119.6327)
  line L1460 (55.364, -119.6327) -> (58.0178, -119.6327)
  line L1461 (58.0178, -119.6327) -> (58.0178, -116.6811)
  line L1462 (58.0178, -116.6811) -> (58.0197, -116.6716)
  line L1463 (58.0197, -116.6716) -> (58.0333, -116.658)
  line L1464 (58.0333, -116.658) -> (58.0428, -116.6561)
  line L1465 (58.0428, -116.6561) -> (60.6968, -116.6561)
  line L1466 (60.6968, -116.6561) -> (60.6968, -115.4905)
  line L1467 (60.6968, -115.4905) -> (60.6987, -115.4809)
  line L1468 (60.6987, -115.4809) -> (60.7123, -115.4674)
  line L1469 (60.7123, -115.4674) -> (60.7218, -115.4655)
  line L1470 (60.7218, -115.4655) -> (67.8656, -115.4655)
  line L1471 (67.8656, -115.4655) -> (67.8751, -115.4674)
  line L1472 (60.7468, -115.5155) -> (60.7468, -116.6811)
  line L1473 (60.7468, -116.6811) -> (60.7449, -116.6907)
  line L1474 (60.7449, -116.6907) -> (60.7314, -116.7042)
  line L1475 (60.7314, -116.7042) -> (60.7218, -116.7061)
  line L1476 (60.7218, -116.7061) -> (58.0678, -116.7061)
  line L1477 (58.0678, -116.7061) -> (58.0678, -119.6577)
  line L1478 (58.0678, -119.6577) -> (58.0659, -119.6673)
  line L1479 (58.0659, -119.6673) -> (58.0524, -119.6808)
  line L1480 (58.0524, -119.6808) -> (58.0428, -119.6827)
  line L1481 (58.0428, -119.6827) -> (55.389, -119.6827)
  line L1482 (55.389, -119.6827) -> (55.389, -125.5858)
  line L1483 (55.389, -125.5858) -> (58.0178, -125.5858)
  line L1484 (58.0178, -125.5858) -> (58.0178, -125.0155)
  line L1485 (58.0178, -125.0155) -> (58.0197, -125.0059)
  line L1486 (58.0197, -125.0059) -> (58.0333, -124.9924)
  line L1487 (58.0333, -124.9924) -> (58.0428, -124.9905)
  line L1488 (58.0428, -124.9905) -> (60.3991, -124.9905)
  line L1489 (60.3991, -124.9905) -> (60.3991, -123.2296)
  line L1490 (60.3991, -123.2296) -> (60.401, -123.22)
  line L1491 (60.401, -123.22) -> (60.4145, -123.2065)
  line L1492 (60.4145, -123.2065) -> (60.4241, -123.2046)
  line L1493 (60.4241, -123.2046) -> (61.9124, -123.2046)
  line L1494 (61.9124, -123.2046) -> (61.9219, -123.2065)
  line L1495 (61.9219, -123.2065) -> (61.9355, -123.22)
  line L1496 (61.9355, -123.22) -> (61.9374, -123.2296)
  line L1497 (61.9374, -123.2296) -> (61.9374, -126.1811)
  line L1498 (61.9374, -126.1811) -> (62.21, -126.1811)
  line L1499 (62.21, -126.1811) -> (66.6499, -126.1811)
  line L1500 (66.6499, -126.1811) -> (66.6499, -125.0155)
  line L1501 (66.6499, -125.0155) -> (66.6499, -121.146)
  line L1502 (66.6499, -121.146) -> (66.6518, -121.1364)
  line L1503 (66.6518, -121.1364) -> (66.6653, -121.1229)
  line L1504 (66.6653, -121.1229) -> (66.6749, -121.121)
  line L1505 (66.6749, -121.121) -> (69.3288, -121.121)
  line L1506 (69.3288, -121.121) -> (69.3288, -120.253)
  line L1507 (69.3288, -120.253) -> (69.3307, -120.2434)
  line L1508 (69.3307, -120.2434) -> (69.3442, -120.2299)
  line L1509 (69.3442, -120.2299) -> (69.3538, -120.228)
  line L1510 (69.3538, -120.228) -> (71.71, -120.228)
  line L1511 (71.71, -120.228) -> (71.71, -116.7061)
  line L1512 (71.71, -116.7061) -> (67.8656, -116.7061)
  line L1513 (67.8656, -116.7061) -> (67.856, -116.7042)
  line L1514 (67.856, -116.7042) -> (67.8425, -116.6907)
  line L1515 (67.8425, -116.6907) -> (67.8425, -116.6907)
  line L1516 (67.8425, -116.6907) -> (67.8406, -116.6811)
  line L1517 (67.8406, -116.6811) -> (67.8406, -115.5155)
  line L1518 (67.8406, -115.5155) -> (60.7468, -115.5155)
  line L1519 (73.2329, -122.3135) -> (73.2465, -122.327)
  line L1520 (73.2465, -122.327) -> (73.2484, -122.3366)
  line L1521 (73.2484, -122.3366) -> (73.2484, -125.3132)
  line L1522 (73.2484, -125.3132) -> (73.2465, -125.3227)
  line L1523 (73.2465, -125.3227) -> (73.2329, -125.3363)
  line L1524 (73.2329, -125.3363) -> (73.2234, -125.3382)
  line L1525 (73.2234, -125.3382) -> (69.3538, -125.3382)
  line L1526 (69.3538, -125.3382) -> (69.1171, -125.3195)
  line L1527 (69.1171, -125.3195) -> (68.8862, -125.2641)
  line L1528 (68.8862, -125.2641) -> (68.6668, -125.1732)
  line L1529 (68.6668, -125.1732) -> (68.4644, -125.0491)
  line L1530 (68.4644, -125.0491) -> (68.2838, -124.8949)
  line L1531 (68.2838, -124.8949) -> (68.1296, -124.7144)
  line L1532 (68.1296, -124.7144) -> (68.0055, -124.5119)
  line L1533 (68.0055, -124.5119) -> (67.9146, -124.2925)
  line L1534 (67.9146, -124.2925) -> (67.8592, -124.0616)
  line L1535 (67.8592, -124.0616) -> (67.8406, -123.8249)
  line L1536 (67.8406, -123.8249) -> (67.8592, -123.5882)
  line L1537 (67.8592, -123.5882) -> (67.9146, -123.3573)
  line L1538 (67.9146, -123.3573) -> (68.0055, -123.1379)
  line L1539 (68.0055, -123.1379) -> (68.1296, -122.9354)
  line L1540 (68.1296, -122.9354) -> (68.2838, -122.7548)
  line L1541 (68.2838, -122.7548) -> (68.4644, -122.6006)
  line L1542 (68.4644, -122.6006) -> (68.6668, -122.4765)
  line L1543 (68.6668, -122.4765) -> (68.8862, -122.3857)
  line L1544 (68.8862, -122.3857) -> (69.1171, -122.3302)
  line L1545 (69.1171, -122.3302) -> (69.3538, -122.3116)
  line L1546 (69.3538, -122.3116) -> (69.3538, -122.3116)
  line L1547 (69.3538, -122.3116) -> (73.2234, -122.3116)
  line L1548 (73.2234, -122.3116) -> (73.2329, -122.3135)
  line L1549 (69.3538, -122.3616) -> (69.3538, -122.3616)
  line L1550 (69.3538, -122.3616) -> (69.2387, -122.3616)
  line L1551 (69.2387, -122.3616) -> (69.0112, -122.3976)
  line L1552 (69.0112, -122.3976) -> (68.7921, -122.4688)
  line L1553 (68.7921, -122.4688) -> (68.5869, -122.5734)
  line L1554 (68.5869, -122.5734) -> (68.4006, -122.7088)
  line L1555 (68.4006, -122.7088) -> (68.2377, -122.8716)
  line L1556 (68.2377, -122.8716) -> (68.1023, -123.058)
  line L1557 (68.1023, -123.058) -> (67.9978, -123.2632)
  line L1558 (67.9978, -123.2632) -> (67.9266, -123.4822)
  line L1559 (67.9266, -123.4822) -> (67.8906, -123.7097)
  line L1560 (67.8906, -123.7097) -> (67.8906, -123.94)
  line L1561 (67.8906, -123.94) -> (67.9266, -124.1675)
  line L1562 (67.9266, -124.1675) -> (67.9978, -124.3866)
  line L1563 (67.9978, -124.3866) -> (68.1023, -124.5918)
  line L1564 (68.1023, -124.5918) -> (68.2377, -124.7781)
  line L1565 (68.2377, -124.7781) -> (68.4006, -124.941)
  line L1566 (68.4006, -124.941) -> (68.5869, -125.0764)
  line L1567 (68.5869, -125.0764) -> (68.7921, -125.181)
  line L1568 (68.7921, -125.181) -> (69.0112, -125.2521)
  line L1569 (69.0112, -125.2521) -> (69.2387, -125.2882)
  line L1570 (69.2387, -125.2882) -> (69.3538, -125.2882)
  line L1571 (69.3538, -125.2882) -> (73.1984, -125.2882)
  line L1572 (73.1984, -125.2882) -> (73.1984, -122.3616)
  line L1573 (73.1984, -122.3616) -> (69.3538, -122.3616)
  line L1574 (88.4346, -113.5269) -> (88.4481, -113.5404)
  line L1575 (88.4481, -113.5404) -> (88.45, -113.55)
  line L1576 (88.45, -113.55) -> (88.45, -115.05)
  line L1577 (88.45, -115.05) -> (88.4481, -115.0596)
  line L1578 (88.4481, -115.0596) -> (88.4346, -115.0731)
  line L1579 (88.4346, -115.0731) -> (88.425, -115.075)
  line L1580 (88.425, -115.075) -> (83.025, -115.075)
  line L1581 (83.025, -115.075) -> (83.0154, -115.0731)
  line L1582 (83.0154, -115.0731) -> (83.0019, -115.0596)
  line L1583 (83.0019, -115.0596) -> (83, -115.05)
  line L1584 (83, -115.05) -> (83, -113.55)
  line L1585 (83, -113.55) -> (83.0019, -113.5404)
  line L1586 (83.0019, -113.5404) -> (83.0154, -113.5269)
  line L1587 (83.0154, -113.5269) -> (83.025, -113.525)
  line L1588 (83.025, -113.525) -> (88.425, -113.525)
  line L1589 (88.425, -113.525) -> (88.4346, -113.5269)
  line L1590 (83.05, -113.575) -> (83.05, -115.025)
  line L1591 (83.05, -115.025) -> (88.4, -115.025)
  line L1592 (88.4, -115.025) -> (88.4, -113.575)
  line L1593 (88.4, -113.575) -> (83.05, -113.575)
  line L1594 (107.4846, -113.5269) -> (107.4981, -113.5404)
  line L1595 (107.4981, -113.5404) -> (107.5, -113.55)
  line L1596 (107.5, -113.55) -> (107.5, -115.05)
  line L1597 (107.5, -115.05) -> (107.4981, -115.0596)
  line L1598 (107.4981, -115.0596) -> (107.4846, -115.0731)
  line L1599 (107.4846, -115.0731) -> (107.475, -115.075)
  line L1600 (107.475, -115.075) -> (102.075, -115.075)
  line L1601 (102.075, -115.075) -> (102.0654, -115.0731)
  line L1602 (102.0654, -115.0731) -> (102.0519, -115.0596)
  line L1603 (102.0519, -115.0596) -> (102.05, -115.05)
  line L1604 (102.05, -115.05) -> (102.05, -113.55)
  line L1605 (102.05, -113.55) -> (102.0519, -113.5404)
  line L1606 (102.0519, -113.5404) -> (102.0654, -113.5269)
  line L1607 (102.0654, -113.5269) -> (102.075, -113.525)
  line L1608 (102.075, -113.525) -> (107.475, -113.525)
  line L1609 (107.475, -113.525) -> (107.4846, -113.5269)
  line L1610 (102.1, -113.575) -> (102.1, -115.025)
  line L1611 (102.1, -115.025) -> (107.45, -115.025)
  line L1612 (107.45, -115.025) -> (107.45, -113.575)
  line L1613 (107.45, -113.575) -> (102.1, -113.575)
  line L1614 (126.5346, -113.5269) -> (126.5481, -113.5404)
  line L1615 (126.5481, -113.5404) -> (126.55, -113.55)
  line L1616 (126.55, -113.55) -> (126.55, -115.05)
  line L1617 (126.55, -115.05) -> (126.5481, -115.0596)
  line L1618 (126.5481, -115.0596) -> (126.5346, -115.0731)
  line L1619 (126.5346, -115.0731) -> (126.525, -115.075)
  line L1620 (126.525, -115.075) -> (121.125, -115.075)
  line L1621 (121.125, -115.075) -> (121.1154, -115.0731)
  line L1622 (121.1154, -115.0731) -> (121.1019, -115.0596)
  line L1623 (121.1019, -115.0596) -> (121.1, -115.05)
  line L1624 (121.1, -115.05) -> (121.1, -113.55)
  line L1625 (121.1, -113.55) -> (121.1019, -113.5404)
  line L1626 (121.1019, -113.5404) -> (121.1154, -113.5269)
  line L1627 (121.1154, -113.5269) -> (121.125, -113.525)
  line L1628 (121.125, -113.525) -> (126.525, -113.525)
  line L1629 (126.525, -113.525) -> (126.5346, -113.5269)
  line L1630 (121.15, -113.575) -> (121.15, -115.025)
  line L1631 (121.15, -115.025) -> (126.5, -115.025)
  line L1632 (126.5, -115.025) -> (126.5, -113.575)
  line L1633 (126.5, -113.575) -> (121.15, -113.575)
  line L1634 (145.5846, -113.5269) -> (145.5981, -113.5404)
  line L1635 (145.5981, -113.5404) -> (145.6, -113.55)
  line L1636 (145.6, -113.55) -> (145.6, -115.05)
  line L1637 (145.6, -115.05) -> (145.5981, -115.0596)
  line L1638 (145.5981, -115.0596) -> (145.5846, -115.0731)
  line L1639 (145.5846, -115.0731) -> (145.575, -115.075)
  line L1640 (145.575, -115.075) -> (140.175, -115.075)
  line L1641 (140.175, -115.075) -> (140.1654, -115.0731)
  line L1642 (140.1654, -115.0731) -> (140.1519, -115.0596)
  line L1643 (140.1519, -115.0596) -> (140.15, -115.05)
  line L1644 (140.15, -115.05) -> (140.15, -113.55)
  line L1645 (140.15, -113.55) -> (140.1519, -113.5404)
  line L1646 (140.1519, -113.5404) -> (140.1654, -113.5269)
  line L1647 (140.1654, -113.5269) -> (140.175, -113.525)
  line L1648 (140.175, -113.525) -> (145.575, -113.525)
  line L1649 (145.575, -113.525) -> (145.5846, -113.5269)
  line L1650 (140.2, -113.575) -> (140.2, -115.025)
  line L1651 (140.2, -115.025) -> (145.55, -115.025)
  line L1652 (145.55, -115.025) -> (145.55, -113.575)
  line L1653 (145.55, -113.575) -> (140.2, -113.575)
  line L1654 (93.1758, -102.3705) -> (93.1894, -102.3841)
  line L1655 (93.1894, -102.3841) -> (93.1913, -102.3936)
  line L1656 (93.1913, -102.3936) -> (93.1913, -105.9655)
  line L1657 (93.1913, -105.9655) -> (93.1894, -105.9751)
  line L1658 (93.1894, -105.9751) -> (93.1758, -105.9886)
  line L1659 (93.1758, -105.9886) -> (93.1663, -105.9905)
  line L1660 (93.1663, -105.9905) -> (90.81, -105.9905)
  line L1661 (90.81, -105.9905) -> (90.81, -106.8585)
  line L1662 (90.81, -106.8585) -> (90.8081, -106.868)
  line L1663 (90.8081, -106.868) -> (90.7946, -106.8816)
  line L1664 (90.7946, -106.8816) -> (90.785, -106.8835)
  line L1665 (90.785, -106.8835) -> (88.1311, -106.8835)
  line L1666 (88.1311, -106.8835) -> (88.1311, -110.728)
  line L1667 (88.1311, -110.728) -> (88.1311, -111.9186)
  line L1668 (88.1311, -111.9186) -> (88.1292, -111.9282)
  line L1669 (88.1292, -111.9282) -> (88.1157, -111.9417)
  line L1670 (88.1157, -111.9417) -> (88.1061, -111.9436)
  line L1671 (88.1061, -111.9436) -> (83.6413, -111.9436)
  line L1672 (83.6413, -111.9436) -> (83.3436, -111.9436)
  line L1673 (83.3436, -111.9436) -> (83.334, -111.9417)
  line L1674 (83.334, -111.9417) -> (83.3205, -111.9282)
  line L1675 (83.3205, -111.9282) -> (83.3186, -111.9186)
  line L1676 (83.3186, -111.9186) -> (83.3186, -108.9671)
  line L1677 (83.3186, -108.9671) -> (81.8803, -108.9671)
  line L1678 (81.8803, -108.9671) -> (81.8803, -110.728)
  line L1679 (81.8803, -110.728) -> (81.8784, -110.7376)
  line L1680 (81.8784, -110.7376) -> (81.8649, -110.7511)
  line L1681 (81.8649, -110.7511) -> (81.8553, -110.753)
  line L1682 (81.8553, -110.753) -> (79.4741, -110.753)
  line L1683 (79.4741, -110.753) -> (79.4645, -110.7511)
  line L1684 (79.4645, -110.7511) -> (79.451, -110.7376)
  line L1685 (79.451, -110.7376) -> (79.4491, -110.728)
  line L1686 (79.4491, -110.728) -> (79.4491, -108.6694)
  line L1687 (79.4491, -108.6694) -> (77.0928, -108.6694)
  line L1688 (77.0928, -108.6694) -> (77.0833, -108.6675)
  line L1689 (77.0833, -108.6675) -> (77.0697, -108.654)
  line L1690 (77.0697, -108.654) -> (77.0678, -108.6444)
  line L1691 (77.0678, -108.6444) -> (77.0678, -105.3702)
  line L1692 (77.0678, -105.3702) -> (77.0697, -105.3606)
  line L1693 (77.0697, -105.3606) -> (77.0833, -105.3471)
  line L1694 (77.0833, -105.3471) -> (77.0928, -105.3452)
  line L1695 (77.0928, -105.3452) -> (79.4491, -105.3452)
  line L1696 (79.4491, -105.3452) -> (79.4491, -102.3936)
  line L1697 (79.4491, -102.3936) -> (79.451, -102.3841)
  line L1698 (79.451, -102.3841) -> (79.4645, -102.3705)
  line L1699 (79.4645, -102.3705) -> (79.4741, -102.3686)
  line L1700 (79.4741, -102.3686) -> (93.1663, -102.3686)
  line L1701 (93.1663, -102.3686) -> (93.1758, -102.3705)
  line L1702 (79.4991, -102.4186) -> (79.4991, -105.3702)
  line L1703 (79.4991, -105.3702) -> (79.4972, -105.3798)
  line L1704 (79.4972, -105.3798) -> (79.4836, -105.3933)
  line L1705 (79.4836, -105.3933) -> (79.4741, -105.3952)
  line L1706 (79.4741, -105.3952) -> (77.1178, -105.3952)
  line L1707 (77.1178, -105.3952) -> (77.1178, -108.6194)
  line L1708 (77.1178, -108.6194) -> (79.4741, -108.6194)
  line L1709 (79.4741, -108.6194) -> (79.4836, -108.6213)
  line L1710 (79.4836, -108.6213) -> (79.4972, -108.6348)
  line L1711 (79.4972, -108.6348) -> (79.4991, -108.6444)
  line L1712 (79.4991, -108.6444) -> (79.4991, -110.703)
  line L1713 (79.4991, -110.703) -> (81.8303, -110.703)
  line L1714 (81.8303, -110.703) -> (81.8303, -108.9421)
  line L1715 (81.8303, -108.9421) -> (81.8322, -108.9325)
  line L1716 (81.8322, -108.9325) -> (81.8458, -108.919)
  line L1717 (81.8458, -108.919) -> (81.8553, -108.9171)
  line L1718 (81.8553, -108.9171) -> (83.3436, -108.9171)
  line L1719 (83.3436, -108.9171) -> (83.3532, -108.919)
  line L1720 (83.3532, -108.919) -> (83.3667, -108.9325)
  line L1721 (83.3667, -108.9325) -> (83.3686, -108.9421)
  line L1722 (83.3686, -108.9421) -> (83.3686, -111.8936)
  line L1723 (83.3686, -111.8936) -> (83.6413, -111.8936)
  line L1724 (83.6413, -111.8936) -> (88.0811, -111.8936)
  line L1725 (88.0811, -111.8936) -> (88.0811, -110.728)
  line L1726 (88.0811, -110.728) -> (88.0811, -106.8585)
  line L1727 (88.0811, -106.8585) -> (88.083, -106.8489)
  line L1728 (88.083, -106.8489) -> (88.0965, -106.8354)
  line L1729 (88.0965, -106.8354) -> (88.1061, -106.8335)
  line L1730 (88.1061, -106.8335) -> (90.76, -106.8335)
  line L1731 (90.76, -106.8335) -> (90.76, -105.9655)
  line L1732 (90.76, -105.9655) -> (90.7619, -105.9559)
  line L1733 (90.7619, -105.9559) -> (90.7754, -105.9424)
  line L1734 (90.7754, -105.9424) -> (90.785, -105.9405)
  line L1735 (90.785, -105.9405) -> (93.1413, -105.9405)